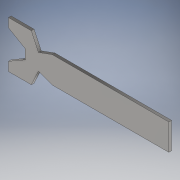
# Autodesk Inventor part: Spare Blade (In Blade Holder)
Saved by Autodesk Inventor 2021 (Build 250183000, 183)
## iProperties
Created: 2021-05-04
Part Number: Spare Blade (In Blade Holder)
Material: Generic
Document SubType Name: Modeling
Designer: AHUJA
Density: 1 g/cm^3
Appearance: Default
Author: AHUJA
Autodesk Inventor part; units mm, degrees
ref_plane "YZ Plane" through (0, 0, 0) normal (1, 0, 0) x (0, 1, 0)
ref_plane "XZ Plane" through (0, 0, 0) normal (0, 1, 0) x (-1, 0, 0)
ref_plane "XY Plane" through (0, 0, 0) normal (0, 0, 1) x (1, 0, 0)
sketch "Sketch1" plane through (0, 0, 0) normal (0, 0, 1) x (1, 0, 0)
  line L0 (0, 0) -> (80, 0)
  line L1 (80, 0) -> (80, 18)
  line L2 (80, 18) -> (0, 18)
  line L3 (0, 18) -> (0, 0)
  line L4 (0, 25) -> (-30, 25)
  line L5 (-30, -7) -> (0, -7)
  line L6 (0, -7) -> (0, 25)
  line L7 (0, 18) -> (-9.3969, 14.5798)
  line L8 (0, 18) -> (10, 18) construction
  line L9 (0, 0) -> (-9.3969, 3.4202)
  line L10 (0, 0) -> (10, 0) construction
  line L11 (-9.3969, 14.5798) -> (-14.2559, 25)
  line L12 (-9.3969, 14.5798) -> (2.1005, 14.5798) construction
  line L13 (-9.3969, 3.4202) -> (-14.2559, -7)
  line L14 (-9.3969, 3.4202) -> (2.1005, 3.4202) construction
  line L15 (-30, 25) -> (-30, 19)
  line L16 (-30, 19) -> (-18.3849, 12.294)
  line L17 (-30, -7) -> (-30, -1)
  line L18 (-30, -1) -> (-18.3849, 5.706)
  line L19 (-18.3849, 5.706) -> (-18.3849, 12.294)
  line L20 (-30, 25) -> (-30, 19)
  line L21 (-30, -1) -> (-30, -7)
  dimension "d0" = 80
  dimension "d1" = 18
  dimension "d2" = 30
  dimension "d3" = 0
  dimension "d4" = 7
  dimension "d5" = 7
  dimension "d6" = 160
  dimension "d7" = 160
  dimension "d8" = 10
  dimension "d9" = 10
  dimension "d10" = 115
  dimension "d11" = 115
  dimension "d12" = 6
  dimension "d13" = 120
  dimension "d14" = 6
  dimension "d15" = 120
  dimension "d16" = 30
  constraints: 44 end point, 6 horizontal, 6 parallel, 4 equal length, 3 perpendicular, 2 point on line
  measures "d0" distance of L1.end L2.end
  measures "d1" distance of L0.end L1.end
  measures "d2" distance of L4.start L4.end
  measures "d3" distance between parallel lines of L3 L6
  measures "d4" distance between parallel lines of L2 L4
  measures "d5" distance between parallel lines of L5 L0
  measures "d6" angle of L7 L8
  measures "d7" angle of L10 L9
  measures "d8" distance of L2.end L7.end
  measures "d9" distance of L0.start L9.end
  measures "d10" angle of L12 L11
  measures "d11" angle of L13 L14
  measures "d12" distance of L4.end L15.end
  measures "d13" angle of L16 L15
  measures "d14" distance of L5.start L17.end
  measures "d15" angle of L17 L18
  measures "d16" distance of L5.start L5.end
extrude "Extrusion1" add sketch "Sketch1" along normal blind 1.905 contours L3 L2 L1 L0 | L9 L13 L5 L17 L18 L19 L16 L15 L4 L11 L7 L3
body "Solid1"
